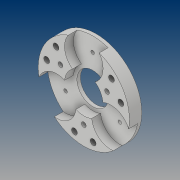
# Autodesk Inventor part: Diskos_Forea1
Saved by Autodesk Inventor 2021 (Build 250183000, 183)
## iProperties
Created: 2020-12-26
Part Number: Diskos_Forea1
Material: Generic
Document SubType Name: Modeling
Designer: Dimitris
Density: 1 g/cm^3
Appearance: Default
Author: Dimitris
Autodesk Inventor part; units mm, degrees
ref_plane "XY Plane" through (0, 0, 0) normal (0, 0, 1) x (1, 0, 0)
sketch "Sketch1" plane through (0, 0, 0) normal (0, 0, 1) x (1, 0, 0)
  circle A0 centre (0, 0) radius 195
  dimension "d0" = 390
  constraints: 1 centre point, 1 coincident
  measures "d0" diameter of A0
extrude "Extrusion1" add sketch "Sketch1" along normal mid plane 53
sketch "Sketch2" plane through (0, 0, 26.5) normal (0, 0, 1) x (1, 0, 0)
  circle A0 centre (0, 133.838) radius 82.5
  point P0 (0, 0)
  dimension "d3" = 133.838
  dimension "d4" = 165
  constraints: 1 centre point, 1 vertical alignment
  measures "d3" distance of point (0, 0) A0.centre
  measures "d4" diameter of A0
extrude "Extrusion2" cut sketch "Sketch2" against normal blind 38
pattern_circular "Circular Pattern1" count 3 over 360 about axis through (0, 0, -10) along (0, 0, 1) of "Extrusion2"
sketch "Sketch3" plane through (0, 0, 26.5) normal (0, 0, 1) x (1, 0, 0)
  circle A0 centre (0, 0) radius 82.5
  dimension "d10" = 165
  constraints: 1 centre point, 1 coincident
  measures "d10" diameter of A0
extrude "Extrusion3" cut sketch "Sketch3" against normal blind 38
sketch "Sketch4" plane through (0, 0, -11.5) normal (0, 0, 1) x (1, 0, 0)
  circle A0 centre (0, 133.838) radius 7.5
  point P0 (0, 0)
  dimension "d13" = 15
  dimension "d14" = 133.838
  constraints: 1 centre point, 1 vertical alignment
  measures "d13" diameter of A0
  measures "d14" distance of A0.centre point (0, 0)
extrude "Extrusion4" cut sketch "Sketch4" against normal through all
pattern_circular "Circular Pattern2" count 3 over 360 about axis through (0, 0, -10) along (0, 0, 1) of "Extrusion4"
sketch "Sketch6" plane through (0, 0, -11.5) normal (0, 0, 1) x (1, 0, 0)
  circle A0 centre (0, 0) radius 67.5
  dimension "d20" = 135
  constraints: 1 centre point, 1 coincident
  measures "d20" diameter of A0
extrude "Extrusion5" cut sketch "Sketch6" against normal through all
sketch "Sketch12" plane through (0, 0, 26.5) normal (0, 0, 1) x (1, 0, 0)
  circle A0 centre (0, -115) radius 10
  point P0 (0, 0)
  dimension "d86" = 20
  dimension "d87" = 115
  constraints: 1 centre point, 1 vertical alignment
  measures "d86" diameter of A0
  measures "d87" distance of point (0, 0) A0.centre
extrude "Extrusion10" cut sketch "Sketch12" against normal through all
pattern_circular "Circular Pattern7" count 3 over 360 about axis through (0, 0, -10) along (0, 0, 1) of "Extrusion10"
sketch "Sketch13" plane through (0, 0, 26.5) normal (0, 0, 1) x (1, 0, 0)
  circle A0 centre (-40, -160) radius 12.5
  circle A1 centre (40, -160) radius 12.5
  point P0 (0, 0)
  dimension "d93" = 25
  dimension "d94" = 40
  dimension "d95" = 160
  dimension "d96" = 25
  dimension "d97" = 40
  dimension "d98" = 160
  constraints: 2 centre point
  measures "d93" diameter of A0
  measures "d94" horizontal distance of point (0, 0) A0.centre
  measures "d95" vertical distance of A0.centre point (0, 0)
  measures "d96" diameter of A1
  measures "d97" horizontal distance of point (0, 0) A1.centre
  measures "d98" vertical distance of point (0, 0) A1.centre
extrude "Extrusion11" cut sketch "Sketch13" against normal blind 40
pattern_circular "Circular Pattern8" count 3 over 360 about axis through (0, 0, -10) along (0, 0, 1) of "Extrusion11"
sketch "Sketch14" plane through (0, 4.875, -26.5) normal (0, 0, -1) x (1, 0, 0)
  arc A0 (1.2533, 9.9211) -> (-1.2533, 9.9211) centre (0, 0) ccw
  arc A1 (0.752, 5.9527) -> (-0.752, 5.9527) centre (0, 0) ccw
  line L0 (-0.752, 5.9527) -> (-1.2533, 9.9211)
  line L1 (0.752, 5.9527) -> (1.2533, 9.9211)
  line L2 (0, 1.5) -> (0, -0.25)
  line L3 (-0.2193, 0) -> (0.2193, 0)
  dimension "d110" = 10
  dimension "d108" = 6
  dimension "d109" = 4
  dimension "d107" = 7.2
  constraints: 8 end point, 4 point on circle, 2 centre point, 2 coincident, 2 horizontal alignment, 1 other
  measures "d110" radius of A0
  measures "d108" radius of A1
  measures "d109" distance of L0.start L0.end
  measures "d107" angle of L2 L0
extrude "Extrusion12" cut sketch "Sketch14" against normal mid plane 80
thread "Thread16" size "M25x2" class "6H" standard "ANSI Metric M Profile" full length
thread "Thread17" size "M25x2" class "6H" standard "ANSI Metric M Profile" full length
thread "Thread18" size "M25x2" class "6H" standard "ANSI Metric M Profile" full length
thread "Thread19" size "M25x2" class "6H" standard "ANSI Metric M Profile" full length
thread "Thread20" size "M25x2" class "6H" standard "ANSI Metric M Profile" full length
thread "Thread21" size "M25x2" class "6H" standard "ANSI Metric M Profile" full length
ref_plane "Work Plane2" through (0, 45.25, 0) normal (0, 1, 0) x (-1, 0, 0)
sketch "Sketch15" plane through (0, 45.25, 0) normal (0, 1, 0) x (-1, 0, 0)
  line L0 (145.8618, -13.3796) -> (158.3612, -13.5)
  line L1 (146.0641, -13.5) -> (171.0641, -13.5) projected
  line L2 (158.3612, -13.5) -> (158.3612, -20.5)
  line L3 (158.3612, -20.5) -> (146.0977, -13.3818)
  point P0 (0, 0)
  point P1 (146.3013, -13.5)
  constraints: 6 end point, 1 perpendicular, 1 point on line
revolve "Revolution1" cut sketch "Sketch15" angle 360 about axis through (-158.3612, 45.25, -13.5) along (0, 0, -1) contours L2 L3 L1
pattern_circular "Circular Pattern9" count 3 over 360 about axis through (0, 0, -11.5) along (0, 0, -1) of "Revolution1"
ref_plane "Work Plane3" through (-118.5, 0, 0) normal (1, 0, 0) x (0, 1, 0)
sketch "Sketch16" plane through (-118.5, 0, 0) normal (1, 0, 0) x (0, 1, 0)
  line L0 (127.141, 26.5) -> (127.141, -13.5) projected
  line L1 (127.141, -13.5) -> (114.641, -13.5)
  line L2 (102.141, -13.5) -> (127.141, -13.5) projected
  line L3 (114.641, -13.5) -> (114.641, -20.5)
  line L4 (114.641, -20.5) -> (127.141, -13.5)
  point P0 (0, 0)
  constraints: 6 end point, 1 collinear, 1 perpendicular, 1 point on line
revolve "Revolution2" cut sketch "Sketch16" angle 360 about axis through (-118.5, 114.641, -13.5) along (0, 0, -1)
pattern_circular "Circular Pattern10" count 3 over 360 about axis through (0, 0, -11.5) along (0, 0, -1) of "Revolution2"
equation "\"d11\" = d5"
equation "\"d14\" = d3"
equation "\"d97\" = d94"
equation "\"d98\" = d95"
equation "\"d110\" = 0.5 * d113"
equation "\"d108\" = -d112 + 0.5 * d113"
equation "\"d109\" = d112"
equation "\"d106\" = d111"
equation "\"d5\" = 38"
equation "\"d113\" = 20"
equation "\"d112\" = 4"
equation "\"d111\" = 80"
body "Solid1"
